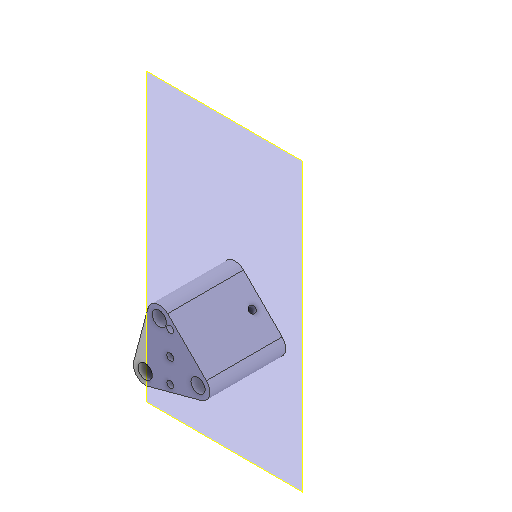
# Autodesk Inventor part: 30_XY_Sample_lightsheetarm_sample_screw_adapter_v3
Saved by Autodesk Inventor 2022 (Build 260153000, 153)
## iProperties
Created: 2021-12-01
Part Number: 30_XY_Sample_lightsheetarm_sample_screw_adapter_v3
Material: Generisch
Document SubType Name: Modeling
Designer: diederichbenedict
Density: 1 g/cm^3
Appearance: Vorgabe
Author: diederichbenedict
Autodesk Inventor part; units mm, degrees
ref_plane "YZ Plane" through (0, 0, 0) normal (1, 0, 0) x (0, 1, 0)
ref_plane "XZ Plane" through (0, 0, 0) normal (0, 1, 0) x (-1, 0, 0)
ref_plane "XY Plane" through (0, 0, 0) normal (0, 0, 1) x (1, 0, 0)
ref_plane "Arbeitsebene1" through (0, 0, -8) normal (0, 0, -1) x (-1, 0, 0)
sketch "Skizze1" plane through (0, 0, -8) normal (0, 0, -1) x (-1, 0, 0)
  line L0 (-30, -73.287606) -> (-18.641556, -61.929162)
  line L1 (-18.641556, -61.929162) -> (-17.580896, -62.989822)
  line L2 (-17.580896, -62.989822) -> (-30, -75.408926)
  line L3 (-30, -75.408926) -> (-30, -76)
  arc A0 (-30, -76) -> (-26, -80) centre (-26, -76) ccw
  line L4 (-18, -80) -> (-26, -80)
  arc A1 (-18, -80) -> (-14, -76) centre (-18, -76) ccw
  line L5 (-14, -34) -> (-14, -76)
  arc A2 (-10, -30) -> (-14, -34) centre (-10, -34) ccw
  line L6 (-10, -30) -> (12, -30)
  arc A3 (16, -34) -> (12, -30) centre (12, -34) ccw
  line L7 (16, -34) -> (16, -76)
  arc A4 (16, -76) -> (20, -80) centre (20, -76) ccw
  line L8 (20, -80) -> (26, -80)
  arc A5 (26, -80) -> (30, -76) centre (26, -76) ccw
  line L9 (30, 28) -> (30, -76)
  line L10 (30, 28) -> (28, 30)
  line L11 (28, 30) -> (-28, 30)
  line L12 (-28, 30) -> (-30, 28)
  line L13 (-30, 28) -> (-30, -73.287606)
  circle A6 centre (-10, -25) radius 1.45
  circle A7 centre (-10, 25) radius 1.45
  circle A8 centre (10, 25) radius 1.45
  circle A9 centre (10, -25) radius 1.45
  circle A10 centre (25, -10) radius 1.45
  circle A11 centre (-25, -10) radius 1.45
  circle A12 centre (-25, 10) radius 1.45
  circle A13 centre (25, 10) radius 1.45
  circle A14 centre (-17.5, -17.5) radius 1.95
  circle A15 centre (17.5, 17.5) radius 1.95
  circle A16 centre (17.5, -17.5) radius 1.95
  circle A17 centre (-17.5, 17.5) radius 1.95
  circle A18 centre (-25, 25) radius 2.325
  circle A19 centre (25, -25) radius 2.325
  circle A20 centre (-25, -25) radius 2.325
  circle A21 centre (25, 25) radius 2.325
  circle A22 centre (0, 0) radius 16
  circle A23 centre (23, -74) radius 3.75
  circle A24 centre (23, -64) radius 1.45
  circle A25 centre (23, -54) radius 1.45
  line L14 (7, -80) -> (39, -80)
  line L15 (39, -80) -> (39, -48)
  line L16 (39, -48) -> (7, -48)
  line L17 (7, -48) -> (7, -80)
  line L18 (7, -80) -> (39, -48) construction
  line L19 (39, -80) -> (7, -48) construction
  circle A26 centre (23, -74) radius 1.4
  line L20 (38.401558, -73.277834) -> (32.4244, -50.970776)
  arc A27 (32.4244, -50.970776) -> (24.059237, -48.729337) centre (27.594771, -52.264871) ccw
  line L21 (24.059237, -48.729337) -> (7.729337, -65.059237)
  arc A28 (7.729337, -65.059237) -> (9.970776, -73.4244) centre (11.264871, -68.594771) ccw
  line L22 (9.970776, -73.4244) -> (32.277834, -79.401558)
  arc A29 (32.277834, -79.401558) -> (38.401558, -73.277834) centre (33.571929, -74.571929) ccw
  circle A30 centre (24.143857, -65.143857) radius 11.666654
  point P0 (0, 0)
  point P1 (26, -80)
  point P2 (30.204536, -48)
  point P3 (16, -48)
  point P4 (16, -56.788574)
  point P5 (7, -65.985006)
  point P6 (7, -71.204536)
  point P7 (19.879318, -76.079386)
  point P8 (24.662897, -77.361142)
  point P9 (24.985006, -48)
  dimension "d0" = 32
  dimension "d1" = 32
  dimension "d2" = 2.8
  constraints: 12 end point, 3 tangent, 2 centre point, 2 midpoint, 2 parallel, 1 coincident, 1 horizontal, 1 perpendicular
  measures "d0" distance of L16.end L15.end
  measures "d1" distance of L15.end L14.end
  measures "d2" diameter of A26
sketch "Skizze1 outline for Extrusion1" plane through (0, 0, -8) normal (0, 0, -1) x (-1, 0, 0)
  line L0 (24.059237, -48.729337) -> (7.729337, -65.059237)
  arc A0 (7.729337, -65.059237) -> (9.970776, -73.4244) centre (11.264871, -68.594771) ccw
  line L1 (9.970776, -73.4244) -> (32.277834, -79.401558)
  arc A1 (32.277834, -79.401558) -> (38.401558, -73.277834) centre (33.571929, -74.571929) ccw
  line L2 (38.401558, -73.277834) -> (32.4244, -50.970776)
  arc A2 (32.4244, -50.970776) -> (24.059237, -48.729337) centre (27.594771, -52.264871) ccw
  circle A3 centre (23, -54) radius 1.45
  circle A4 centre (23, -74) radius 1.4
  circle A5 centre (23, -64) radius 1.45
extrude "Extrusion1" add sketch "Skizze1 outline for Extrusion1" along normal blind 32
sketch "Skizze2" plane through (0, 0, -8) normal (0, 0, -1) x (-1, 0, 0)
  circle A0 centre (33.571929, -74.571929) radius 1.4
  line L0 (33.571929, -74.571929) -> (11.264871, -68.594771)
  line L1 (11.264871, -68.594771) -> (27.594771, -52.264871)
  line L2 (27.594771, -52.264871) -> (33.571929, -74.571929)
  line L3 (9.702889, -90.642573) -> (49.480711, -50.864751) construction
  line L4 (-4.702878, -89.491992) -> (48.33013, -36.458983) construction
  line L5 (39, -80) -> (39, -48) construction
  line L6 (7, -48) -> (7, -80) construction
  line L7 (39, -80) -> (7, -48) construction
  arc A1 (32.4244, -50.970776) -> (24.059237, -48.729337) centre (27.594771, -52.264871) ccw
  line L8 (24.059237, -48.729337) -> (7.729337, -65.059237)
  arc A2 (7.729337, -65.059237) -> (9.970776, -73.4244) centre (11.264871, -68.594771) ccw
  line L9 (9.970776, -73.4244) -> (32.277834, -79.401558)
  arc A3 (32.277834, -79.401558) -> (38.401558, -73.277834) centre (33.571929, -74.571929) ccw
  line L10 (38.401558, -73.277834) -> (32.4244, -50.970776)
  point P0 (0, 0)
  point P1 (24.429821, -55.429821)
  point P2 (24.143857, -65.143857)
  constraints: 8 end point, 2 point on line, 1 centre point, 1 parallel, 5 other
hole "Bohrung1" at (-27.594771, -52.264871, -8) at (-11.264871, -68.594771, -8) at (-33.571929, -74.571929, -8) direction (0, 0, -1) diameter 2.8 end through all counterbore diameter 6 counterbore depth 25
sketch "Skizze4" plane through (-32.4244, -50.970776, -40) normal (-0.9659258, 0.258819, 0) x (0, 0, 1)
  line L0 (6.9, -13.046983) -> (-22.693275, -13.046983)
  line L1 (6.9, -10.046983) -> (-22.693275, -10.046983)
  circle A0 centre (4.520748, -11.521219) radius 1.4
  point P0 (40, 57.626041)
  dimension "d19" = 2.8
  constraints: 4 end point, 2 horizontal, 1 centre point, 4 other
  measures "d19" diameter of A0
sketch "Skizze4 outline for Extrusion3" plane through (-32.4244, -50.970776, -40) normal (-0.9659258, 0.258819, 0) x (0, 0, 1)
  circle A0 centre (4.520748, -11.521219) radius 1.4
extrude "Extrusion3" cut sketch "Skizze4 outline for Extrusion3" against normal blind 15
sketch "Skizze5" plane through (0, 0, -40) normal (0, 0, -1) x (-1, 0, 0)
  line L0 (9.970776, -73.4244) -> (32.277834, -79.401558)
  line L1 (24.059237, -48.729337) -> (7.729337, -65.059237)
  line L2 (38.401558, -73.277834) -> (32.4244, -50.970776)
  circle A0 centre (24.143857, -65.143857) radius 11.666654
  circle A1 centre (24.143857, -65.143857) radius 0.5
  point P0 (0, 0)
  dimension "d22" = 1
  constraints: 3 tangent, 2 centre point, 1 coincident
  measures "d22" diameter of A1
sketch "Skizze5 outline for Extrusion4" plane through (0, 0, -40) normal (0, 0, -1) x (-1, 0, 0)
  circle A0 centre (24.143857, -65.143857) radius 0.5
extrude "Extrusion4" cut sketch "Skizze5 outline for Extrusion4" against normal blind 1
pattern_circular "Runde Anordnung2" count 3 over 360 about axis through (-24.143857, -65.143857, -40) along (0, 0, 1) of "Extrusion3"
